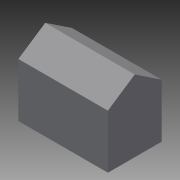
# Autodesk Inventor part: 简单房
Saved by Autodesk Inventor 2015 (Build 190159000, 159)
## iProperties
Created: 2016-07-11
Part Number: 简单房
Material: 常规
Document SubType Name: Modeling
Designer: Administrator
Density: 1 g/cm^3
Appearance: 默认
Author: Administrator
Autodesk Inventor part; units mm, degrees
ref_plane "YZ Plane" through (0, 0, 0) normal (1, 0, 0) x (0, 1, 0)
ref_plane "XZ Plane" through (0, 0, 0) normal (0, 1, 0) x (-1, 0, 0)
ref_plane "XY Plane" through (0, 0, 0) normal (0, 0, 1) x (1, 0, 0)
sketch "草图1" plane through (0, 0, 0) normal (0, 0, 1) x (1, 0, 0)
  line L0 (-2500, 1500) -> (2500, 1500)
  line L1 (2500, 1500) -> (2500, -1500)
  line L2 (2500, -1500) -> (-2500, -1500)
  line L3 (-2500, -1500) -> (-2500, 1500)
  point P0 (0, 0)
  point P1 (2500, 0)
  point P2 (0, 1500)
  dimension "d0" = 5000
  dimension "d1" = 3000
  constraints: 8 end point, 2 midpoint, 2 parallel, 1 horizontal, 1 horizontal alignment, 1 perpendicular, 1 vertical alignment
  measures "d0" distance between parallel lines of L1 L3
  measures "d1" distance of L0.end L1.end
extrude "拉伸1" add sketch "草图1" along normal blind 4000
sketch "草图2" plane through (2500, -1500, 0) normal (1, 0, 0) x (0, 0, -1)
  line L0 (-4000, 3000) -> (-4000, 0) projected
  line L1 (-4000, 1500) -> (-3000, 3000)
  line L2 (0, 3000) -> (-4000, 3000) projected
  line L3 (-4000, 1500) -> (-3000, 0)
  line L4 (0, 0) -> (-4000, 0) projected
  line L5 (-3000, 3000) -> (0, 3000)
  line L6 (0, 0) -> (-3000, 0)
  line L7 (0, 3000) -> (0, 0)
  point P0 (0, 1500)
  dimension "d4" = 1000
  constraints: 10 end point, 2 point on line, 1 collinear, 1 horizontal, 1 midpoint, 1 vertical, 1 vertical alignment
  measures "d4" distance from line of L1.end L0
extrude "拉伸2" cut sketch "草图2" against normal through all contours L1 L2 L7 L4 L3 keep common part
